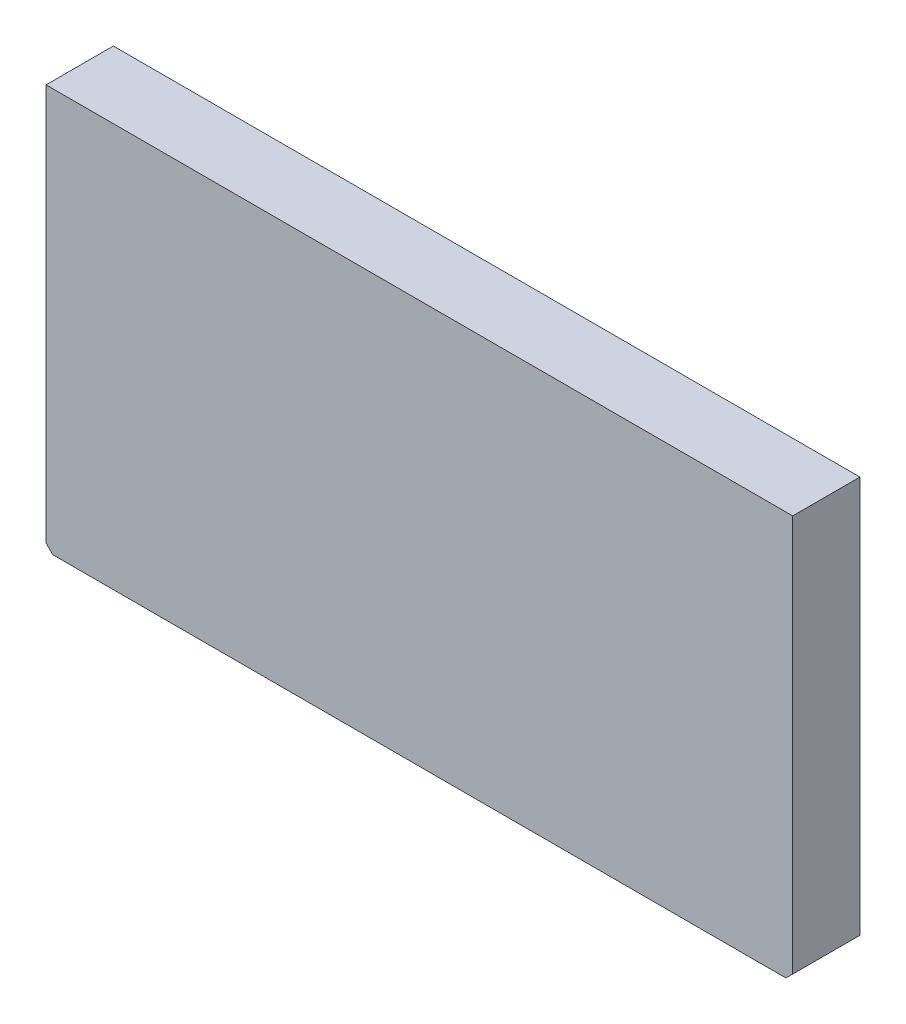
# Autodesk Inventor part: SW_SM_PUSHB
Saved by Autodesk Inventor 2015 SP1 (Build 190203100, 203)
## iProperties
Created: 2015-06-25
Part Number: SW_SM_PUSHB
Material: Generic
Document SubType Name: Modeling
Designer: Patrick
Density: 1 g/cm^3
Appearance: PCBSW_SMT, SW_SM_PUSHB
Author: Patrick
Autodesk Inventor part; units mm, degrees
ref_plane "YZ Plane" through (0, 0, 0) normal (1, 0, 0) x (0, 1, 0)
ref_plane "XZ Plane" through (0, 0, 0) normal (0, 1, 0) x (-1, 0, 0)
ref_plane "XY Plane" through (0, 0, 0) normal (0, 0, 1) x (1, 0, 0)
sketch "PCBSW_SMT, SW_SM_PUSHB_257" plane through (0, 0, 0) normal (0, 0, 1) x (1, 0, 0)
  line L0 (-5.6, 3) -> (5.5, 3)
  line L1 (5.5, 3) -> (5.5, -2.9)
  line L2 (5.5, -2.9) -> (5.4, -3)
  line L3 (5.4, -3) -> (-5.5, -3)
  line L4 (-5.5, -3) -> (-5.6, -2.9)
  line L5 (-5.6, -2.9) -> (-5.6, 3)
  constraints: 12 end point
extrude "Extrusion1" add sketch "PCBSW_SMT, SW_SM_PUSHB_257" along normal blind 1
body "Solid1"
